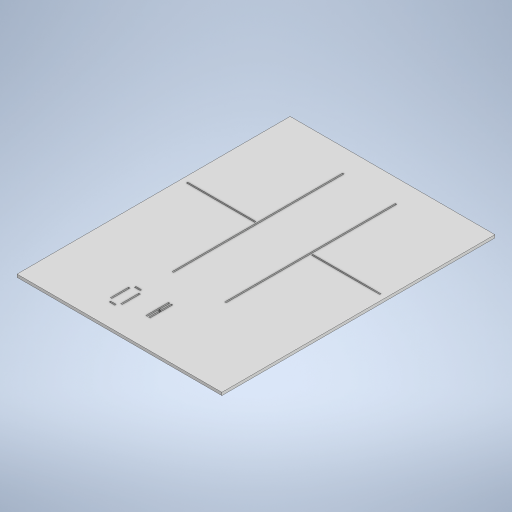
# Autodesk Inventor part: base
Saved by Autodesk Inventor 2023 (Build 270158000, 158)
## iProperties
Created: 2023-10-15
Part Number: base
Material: Generic
Document SubType Name: Modeling
Designer: Nate
Density: 1 g/cm^3
Appearance: Default
Author: Nate
Autodesk Inventor part; units mm, degrees
ref_plane "YZ Plane" through (0, 0, 0) normal (1, 0, 0) x (0, 1, 0)
ref_plane "XZ Plane" through (0, 0, 0) normal (0, 1, 0) x (-1, 0, 0)
ref_plane "XY Plane" through (0, 0, 0) normal (0, 0, 1) x (1, 0, 0)
sketch "Sketch1" plane through (0, 0, 0) normal (0, 1, 0) x (-1, 0, 0)
  line L0 (0, 0) -> (-457.2, 0)
  line L1 (-457.2, 0) -> (-457.2, -609.6)
  line L2 (-457.2, -609.6) -> (0, -609.6)
  line L3 (0, -609.6) -> (0, 0)
  line L4 (-168.275, -558.8) -> (-171.45, -558.8)
  line L5 (-171.45, -558.8) -> (-171.45, -177.8)
  line L6 (-171.45, -177.8) -> (-168.275, -177.8)
  line L7 (-168.275, -177.8) -> (-168.275, -558.8)
  line L8 (-285.75, -558.8) -> (-288.925, -558.8)
  line L9 (-288.925, -558.8) -> (-288.925, -177.8)
  line L10 (-288.925, -177.8) -> (-285.75, -177.8)
  line L11 (-285.75, -177.8) -> (-285.75, -558.8)
  line L12 (-12.7, -368.3) -> (-165.1, -368.3)
  line L13 (-165.1, -368.3) -> (-165.1, -365.125)
  line L14 (-165.1, -365.125) -> (-12.7, -365.125)
  line L15 (-12.7, -365.125) -> (-12.7, -368.3)
  line L16 (-292.1, -368.3) -> (-444.5, -368.3)
  line L17 (-444.5, -368.3) -> (-444.5, -365.125)
  line L18 (-444.5, -365.125) -> (-292.1, -365.125)
  line L19 (-292.1, -365.125) -> (-292.1, -368.3)
  line L20 (-223.8375, -63.5) -> (-227.0125, -63.5)
  line L21 (-227.0125, -63.5) -> (-227.0125, -114.3)
  line L22 (-227.0125, -114.3) -> (-223.8375, -114.3)
  line L23 (-223.8375, -114.3) -> (-223.8375, -63.5)
  line L24 (-230.1875, -63.5) -> (-233.3625, -63.5)
  line L25 (-233.3625, -63.5) -> (-233.3625, -114.3)
  line L26 (-233.3625, -114.3) -> (-230.1875, -114.3)
  line L27 (-230.1875, -114.3) -> (-230.1875, -63.5)
  line L28 (-153.0477, -105.5116) -> (-173.0375, -105.5116)
  line L29 (-173.0375, -105.5116) -> (-173.0375, -52.07)
  line L30 (-173.0375, -52.07) -> (-153.0477, -52.07)
  line L31 (-153.0477, -52.07) -> (-153.0477, -105.5116)
  line L32 (-156.6926, -105.5116) -> (-169.3926, -105.5116)
  line L33 (-169.3926, -105.5116) -> (-169.3926, -108.6866)
  line L34 (-169.3926, -108.6866) -> (-156.6926, -108.6866)
  line L35 (-156.6926, -108.6866) -> (-156.6926, -105.5116)
  line L36 (-156.6926, -52.07) -> (-169.3926, -52.07)
  line L37 (-169.3926, -52.07) -> (-169.3926, -48.895)
  line L38 (-169.3926, -48.895) -> (-156.6926, -48.895)
  line L39 (-156.6926, -48.895) -> (-156.6926, -52.07)
  line L40 (-153.0477, -99.1108) -> (-149.8727, -99.1108)
  line L41 (-149.8727, -99.1108) -> (-149.8727, -58.4708)
  line L42 (-149.8727, -58.4708) -> (-153.0477, -58.4708)
  line L43 (-153.0477, -58.4708) -> (-153.0477, -99.1108)
  line L44 (-173.0375, -58.4708) -> (-176.2125, -58.4708)
  line L45 (-176.2125, -58.4708) -> (-176.2125, -99.1108)
  line L46 (-176.2125, -99.1108) -> (-173.0375, -99.1108)
  line L47 (-173.0375, -99.1108) -> (-173.0375, -58.4708)
  line L48 (-227.0125, -87.3125) -> (-230.1875, -87.3125)
  line L49 (-230.1875, -87.3125) -> (-230.1875, -90.4875)
  line L50 (-230.1875, -90.4875) -> (-227.0125, -90.4875)
  line L51 (-227.0125, -90.4875) -> (-227.0125, -87.3125)
  point P0 (-169.8625, -558.8)
  point P1 (-169.8625, -177.8)
  point P2 (-287.3375, -558.8)
  point P3 (-287.3375, -177.8)
  point P4 (-168.275, -368.3)
  point P5 (-165.1, -366.7125)
  point P6 (-292.1, -366.7125)
  point P7 (-225.425, -63.5)
  point P8 (-163.0426, -105.5116)
  point P9 (-156.6926, -107.0991)
  point P10 (-156.6926, -50.4825)
  point P11 (-151.4602, -99.1108)
  point P12 (-169.3926, -105.5116)
  dimension "d0" = 457.2
  dimension "d1" = 609.6
  dimension "d2" = 3.175
  dimension "d3" = 3.175
  dimension "d4" = 381
  dimension "d5" = 381
  dimension "d6" = 50.8
  dimension "d7" = 50.8
  dimension "d8" = 114.3
  dimension "d9" = 168.275
  dimension "d10" = 152.4
  dimension "d11" = 3.175
  dimension "d12" = 241.3
  dimension "d13" = 3.175
  dimension "d14" = 152.4
  dimension "d15" = 3.175
  dimension "d16" = 3.175
  dimension "d17" = 241.3
  dimension "d18" = 3.175
  dimension "d19" = 50.8
  dimension "d20" = 3.175
  dimension "d21" = 50.8
  dimension "d22" = 3.175
  dimension "d23" = 223.8375
  dimension "d24" = 19.9898
  dimension "d25" = 53.4416
  dimension "d26" = 50.8
  dimension "d27" = 63.5
  dimension "d29" = 105.5116
  dimension "d30" = 12.7
  dimension "d31" = 3.175
  dimension "d32" = 3.6449
  dimension "d33" = 12.7
  dimension "d34" = 3.175
  dimension "d35" = 3.6449
  dimension "d36" = 3.175
  dimension "d37" = 40.64
  dimension "d38" = 6.4008
  dimension "d39" = 3.175
  dimension "d40" = 40.64
  dimension "d41" = 6.4008
  dimension "d44" = 3.175
  dimension "d45" = 3.175
  dimension "d46" = 23.8125
  constraints: 104 end point, 26 parallel, 13 horizontal, 13 perpendicular, 12 midpoint, 6 point on line
  measures "d0" distance of L2.end L1.end
  measures "d1" distance of L1.end L0.end
  measures "d2" distance of L5.end L6.end
  measures "d3" distance of L9.end L10.end
  measures "d4" distance of point (-169.862, -558.8) point (-169.863, -177.8)
  measures "d5" distance of point (-287.337, -558.8) point (-287.338, -177.8)
  measures "d6" distance from line of L2 point (-169.862, -558.8)
  measures "d7" distance between parallel lines of L2 L8
  measures "d8" distance between parallel lines of L11 L5
  measures "d9" distance between parallel lines of L7 L3
  measures "d10" distance of L13.end L14.end
  measures "d11" distance between parallel lines of L12 L14
  measures "d12" distance between parallel lines of L2 L12
  measures "d13" horizontal distance of point (-168.275, -368.3) point (-165.1, -366.713)
  measures "d14" distance of L17.end L18.end
  measures "d15" distance between parallel lines of L16 L18
  measures "d16" distance from line of L9 point (-292.1, -366.713)
  measures "d17" distance between parallel lines of L2 L16
  measures "d18" distance of L22.end L21.end
  measures "d19" distance of L21.end L20.end
  measures "d20" distance of L26.end L25.end
  measures "d21" distance of L25.end L24.end
  measures "d22" distance between parallel lines of L27 L21
  measures "d23" distance between parallel lines of L3 L23
  measures "d24" distance of L29.end L30.end
  measures "d25" distance of L28.end L29.end
  measures "d26" distance between parallel lines of L23 L29
  measures "d27" distance from line of L0 point (-225.425, -63.5)
  measures "d29" distance from line of L0 point (-163.043, -105.512)
  measures "d30" distance of L34.end L33.end
  measures "d31" distance between parallel lines of L34 L32
  measures "d32" distance from line of point (-156.693, -107.099) L31
  measures "d33" distance of L37.end L38.end
  measures "d34" distance of L36.end L37.end
  measures "d35" distance from line of L31 point (-156.693, -50.482)
  measures "d36" distance of L42.end L41.end
  measures "d37" distance of L41.end L40.end
  measures "d38" distance from line of L28 point (-151.46, -99.111)
  measures "d39" distance of L46.end L45.end
  measures "d40" distance between parallel lines of L46 L44
  measures "d41" distance between parallel lines of L28 L46
  measures "d44" distance of L50.end L49.end
  measures "d45" distance of L49.end L48.end
  measures "d46" distance between parallel lines of L20 L48
extrude "Extrusion1" add sketch "Sketch1" along normal blind 6.35 contours L3 L2 L1 L0 | L28 L29 L30 L31
body "Solid1"
